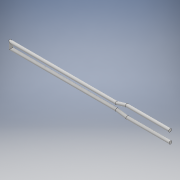
# Autodesk Inventor part: Alambre
Saved by Autodesk Inventor 2017 (Build 210142000, 142)
## iProperties
Created: 2021-07-26
Part Number: Alambre
Material: Generic
Document SubType Name: Modeling
Designer: USUARIO
Density: 1 g/cm^3
Appearance: Default
Author: USUARIO
Autodesk Inventor part; units mm, degrees
ref_plane "YZ Plane" through (0, 0, 0) normal (1, 0, 0) x (0, 1, 0)
ref_plane "XZ Plane" through (0, 0, 0) normal (0, 1, 0) x (-1, 0, 0)
sketch "Sketch1" plane through (0, 0, 0) normal (0, 1, 0) x (-1, 0, 0)
  line L0 (0, 0) -> (110, 0)
  line L1 (110, 0) -> (110, -6)
  line L2 (110, -6) -> (0, -6)
  line L3 (0, -6) -> (-10.8842, -7.5918)
  line L4 (-10.8842, -7.5918) -> (-55.8842, -7.5918)
  line L5 (0, 0) -> (-10.5372, 3.1572)
  line L6 (-10.5372, 3.1572) -> (-55.5372, 3.1572)
  dimension "d0" = 110
  dimension "d1" = 6
  dimension "d2" = 110
  dimension "d3" = 11
  dimension "d4" = 45
  dimension "d5" = 11
  dimension "d6" = 45
  dimension "d10" = 25
  constraints: 14 end point, 3 horizontal, 2 perpendicular
  measures "d0" distance of L0.start L0.end
  measures "d1" distance of L0.end L1.end
  measures "d2" distance of L1.end L2.end
  measures "d3" distance of L2.end L3.end
  measures "d4" distance of L3.end L4.end
  measures "d5" distance of L0.start L5.end
  measures "d6" distance of L5.end L6.end
  measures "d10" angle of L3 L5
ref_plane "Work Plane1" through (55.5372, 0, 3.1572) normal (1, 0, 0) x (0, 1, 0)
sketch "Sketch2" plane through (55.5372, 0, 3.1572) normal (1, 0, 0) x (0, 1, 0)
  circle A0 centre (0, 0) radius 1.5
  point P0 (0, -3.1572)
  dimension "d7" = 3
  constraints: 1 centre point
  measures "d7" diameter of A0
sweep "Sweep1" add profiles "Sketch2" path "Sketch1"
body "Solid1"
